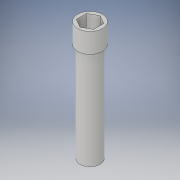
# Autodesk Inventor part: Bolt 13_64 Representation
Saved by Autodesk Inventor 2018 (Build 220112000, 112)
## iProperties
Created: 2018-12-23
Part Number: Bolt 13_64 Representation
Material: Generic
Document SubType Name: Modeling
Designer: Gabriel
Density: 1 g/cm^3
Appearance: Default
Author: Gabriel
Autodesk Inventor part; units mm, degrees
ref_plane "YZ Plane" through (0, 0, 0) normal (1, 0, 0) x (0, 1, 0)
ref_plane "XZ Plane" through (0, 0, 0) normal (0, 1, 0) x (-1, 0, 0)
ref_plane "XY Plane" through (0, 0, 0) normal (0, 0, 1) x (1, 0, 0)
sketch "Sketch1" plane through (0, 0, 0) normal (0, 1, 0) x (-1, 0, 0)
  circle A0 centre (3.5103, 7.6377) radius 2.5797
  point P0 (0, 0)
  dimension "d0" = 5.1594
  constraints: 1 centre point
  measures "d0" diameter of A0
extrude "Extrusion1" add sketch "Sketch1" along normal blind 25.4
sketch "Sketch2" plane through (-3.5103, 25.4, 7.6377) normal (0, 1, 0) x (1, 0, 0)
  circle A0 centre (0, 0) radius 3.175
  point P0 (3.5103, 7.6377)
  dimension "d3" = 6.35
  constraints: 1 centre point
  measures "d3" diameter of A0
extrude "Extrusion2" add sketch "Sketch2" along normal blind 5.08
sketch "Sketch3" plane through (-3.5103, 30.48, 7.6377) normal (0, 1, 0) x (1, 0, 0)
  circle A0 centre (0, 0) radius 2.5797 projected
  line L0 (2.231, 1.2951) -> (2.2371, -1.2846)
  line L1 (2.2371, -1.2846) -> (0.006, -2.5797)
  line L2 (0.006, -2.5797) -> (-2.231, -1.2951)
  line L3 (-2.231, -1.2951) -> (-2.2371, 1.2846)
  line L4 (-2.2371, 1.2846) -> (-0.006, 2.5797)
  line L5 (-0.006, 2.5797) -> (2.231, 1.2951)
  point P0 (3.5103, 7.6377)
  constraints: 12 end point, 15 other
extrude "Extrusion3" cut sketch "Sketch3" against normal blind 3.81 contours L0 L1 L2 L3 L4 L5
body "Solid1"
